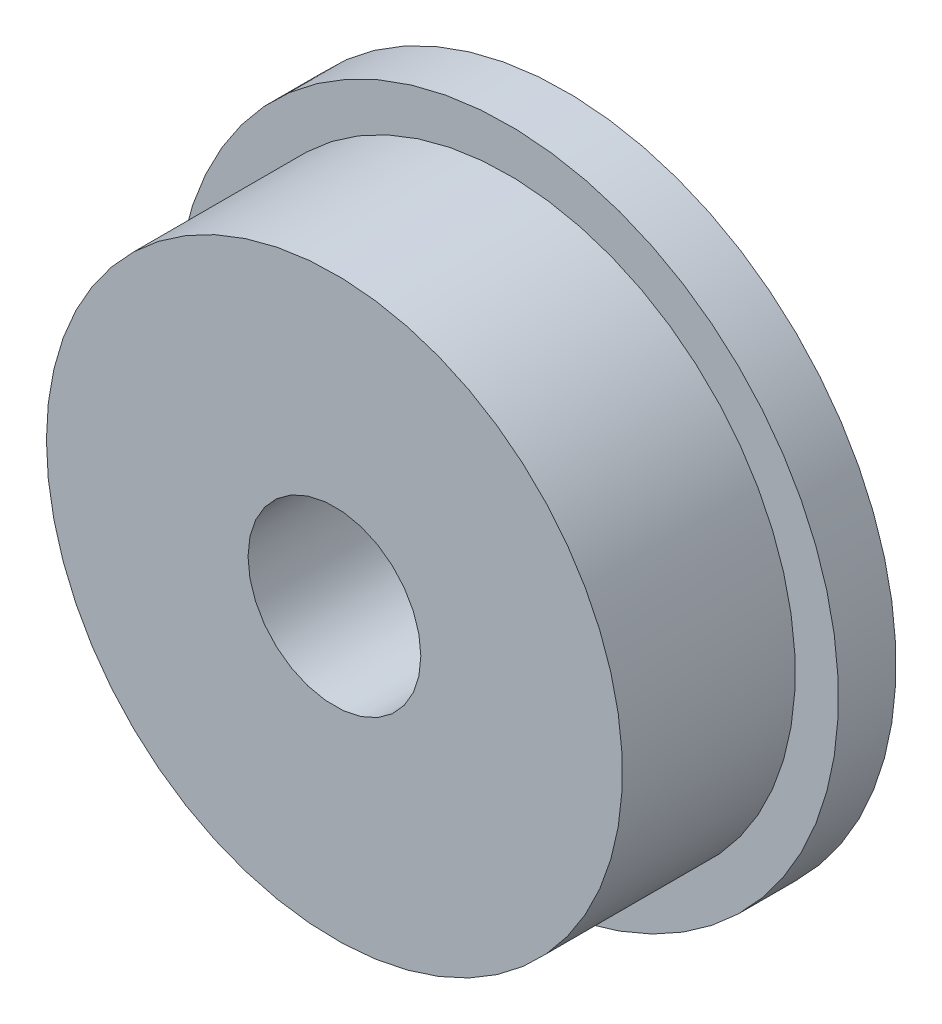
# Autodesk Inventor part: bearing_3x4x10
Saved by Autodesk Inventor 2017.2 (Build 212233000, 233)
## iProperties
Created: 2017-09-03
Part Number: bearing_3x4x10
Material: Generic
Document SubType Name: Modeling
Designer: Nic
Density: 1 g/cm^3
Appearance: Default
Author: Nic
Autodesk Inventor part; units mm, degrees
ref_plane "YZ Plane" through (0, 0, 0) normal (1, 0, 0) x (0, 1, 0)
ref_plane "XZ Plane" through (0, 0, 0) normal (0, 1, 0) x (-1, 0, 0)
ref_plane "XY Plane" through (0, 0, 0) normal (0, 0, 1) x (1, 0, 0)
sketch "Sketch1" plane through (0, 0, 0) normal (0, 1, 0) x (-1, 0, 0)
  line L0 (0, 0) -> (0, 6.5) construction
  line L1 (1.5, 0) -> (5.75, 0)
  line L2 (5.75, 0) -> (5.75, 1)
  line L3 (5.75, 1) -> (5, 1)
  line L4 (5, 1) -> (5, 4)
  line L5 (5, 4) -> (1.5, 4)
  line L6 (1.5, 4) -> (1.5, 0)
  dimension "d0" = 1.5
  dimension "d1" = 5
  dimension "d2" = 4
  dimension "d3" = 1
  dimension "d4" = 0.75
  constraints: 14 end point, 5 perpendicular, 1 horizontal, 1 point on line, 1 vertical
  measures "d0" distance between parallel lines of L0 L6
  measures "d1" distance between parallel lines of L0 L4
  measures "d2" distance between parallel lines of L1 L5
  measures "d3" distance between parallel lines of L1 L3
  measures "d4" distance between parallel lines of L4 L2
revolve "Revolution1" add sketch "Sketch1" angle 360 about axis through (0, 0, 0) along (0, 0, 1)
body "Solid1"
